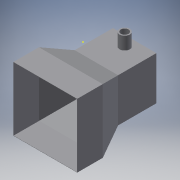
# Autodesk Inventor part: my_subsystem
Saved by Autodesk Inventor 2019 (Build 230136000, 136)
## iProperties
Created: 2020-02-19
Part Number: my_subsystem
Material: Generic
Document SubType Name: Modeling
Designer: Chirag
Density: 1 g/cm^3
Appearance: Default
Author: Chirag
Autodesk Inventor part; units mm, degrees
ref_plane "YZ Plane" through (0, 0, 0) normal (1, 0, 0) x (0, 1, 0)
ref_plane "XZ Plane" through (0, 0, 0) normal (0, 1, 0) x (-1, 0, 0)
ref_plane "XY Plane" through (0, 0, 0) normal (0, 0, 1) x (1, 0, 0)
sketch "Sketch1" plane through (0, 0, 0) normal (0, 0, 1) x (1, 0, 0)
  line L0 (0, 0) -> (250, 0)
  line L1 (250, 0) -> (250, 250)
  line L2 (250, 250) -> (0, 250)
  line L3 (0, 250) -> (0, 0)
  dimension "d0" = 250
  dimension "d1" = 250
  constraints: 8 end point, 2 parallel, 1 horizontal, 1 perpendicular
  measures "d0" distance of L2.end L1.end
  measures "d1" distance of L1.end L0.end
extrude "Extrusion1" add sketch "Sketch1" along normal blind 200
chamfer "Chamfer1" distance 100 distance2 40 1 edges at (0, 125, 0) measured on face at (0, 166.6667, 66.6667)
chamfer "Chamfer2" distance 100 distance2 40 1 edges at (145, 0, 0) measured on face at (180, 0, 66.6667)
chamfer "Chamfer3" distance 100 distance2 40 1 edges at (145, 250, 0) measured on face at (180, 250, 66.6667)
chamfer "Chamfer4" distance 100 distance2 40 1 edges at (250, 125, 0) measured on face at (250, 166.6667, 133.3333)
sketch "Sketch2" plane through (0, 0, 0) normal (0, 0, -1) x (-1, 0, 0)
  line L0 (-40, 40) -> (-210, 40) projected
  line L1 (-210, 210) -> (-40, 210) projected
  line L2 (-40, 40) -> (-210, 40)
  line L3 (-210, 40) -> (-210, 210)
  line L4 (-210, 210) -> (-40, 210)
  line L5 (-40, 210) -> (-40, 40)
  point P0 (0, 0)
  constraints: 8 end point, 2 parallel, 1 horizontal, 1 perpendicular
extrude "Extrusion2" add sketch "Sketch2" along normal blind 150
sketch "Sketch3" plane through (40, 210, 0) normal (0, 1, 0) x (1, 0, 0)
  circle A0 centre (85, 110.8002) radius 20
  point P0 (-40, 0)
  dimension "d18" = 40
  constraints: 1 centre point
  measures "d18" diameter of A0
extrude "Extrusion3" add sketch "Sketch3" along normal blind 50
sketch "Sketch4" plane through (125, 260, -110.8002) normal (0, 1, 0) x (1, 0, 0)
  circle A0 centre (0, 0) radius 15
  point P0 (-125, -110.8002)
  dimension "d21" = 30
  constraints: 1 centre point
  measures "d21" diameter of A0
shell "Shell1" thickness 1 removed faces 1 at (83.3333, 166.6667, 200)
extrude "Extrusion4" cut sketch "Sketch4" against normal blind 60
sketch "Sketch5" plane through (40, 210, 0) normal (0, 1, 0) x (1, 0, 0)
  circle A0 centre (49.0593, 110.2763) radius 5
  point P0 (-40, 0)
  dimension "d25" = 10
  constraints: 1 centre point
  measures "d25" diameter of A0
extrude "Extrusion5" [suppressed]
sketch "Sketch6" plane through (89.0593, 290, -110.2763) normal (0, 1, 0) x (1, 0, 0)
  circle A0 centre (0, 0) radius 5 projected
  line L0 (-5, 0) -> (5, 0)
  line L1 (5, 0) -> (5, -80.1533)
  line L2 (5, -80.1533) -> (-5, -80.1533)
  line L3 (-5, -80.1533) -> (-5, 0)
  point P0 (-89.0593, -110.2763)
  constraints: 8 end point, 2 parallel, 1 horizontal, 1 horizontal alignment, 1 perpendicular, 1 other
extrude "Extrusion6" [suppressed]
sketch "Sketch7" plane through (0, 250, 100) normal (0, 0.9285, -0.3714) x (1, 0, 0)
  point P0 (0, 185.6953)
body "Solid1"
